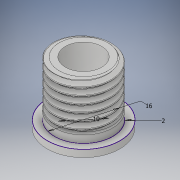
# Autodesk Inventor part: LegScrew
Saved by Autodesk Inventor 2018.2 (Build 222227000, 227)
## iProperties
Created: 2018-03-10
Part Number: LegScrew
Material: Generisch
Document SubType Name: Modeling
Designer: JochenAlt
Density: 1 g/cm^3
Appearance: Vorgabe
Author: JochenAlt
Autodesk Inventor part; units mm, degrees
ref_plane "YZ Plane" through (0, 0, 0) normal (1, 0, 0) x (0, 1, 0)
ref_plane "XZ Plane" through (0, 0, 0) normal (0, 1, 0) x (-1, 0, 0)
ref_plane "XY Plane" through (0, 0, 0) normal (0, 0, 1) x (1, 0, 0)
sketch "Skizze1" plane through (0, 0, 0) normal (0, 0, 1) x (1, 0, 0)
  circle A0 centre (0, 0) radius 5
  circle A1 centre (0, 0) radius 10
  circle A2 centre (0, 0) radius 8
  dimension "d0" = 10
  dimension "d1" = 16
  dimension "d2" = 2
  constraints: 3 centre point, 3 coincident
  measures "d0" diameter of A0
  measures "d1" diameter of A2
  measures "d2" radial gap between concentric circles of A1 A2
extrude "Extrusion1" add sketch "Skizze1" along normal blind 15 contours A2
extrude "Extrusion2" add sketch "Skizze1" against normal blind 2 contours A1 | A2
thread "Gewinde3" size "M16x2" class "6g" standard "ANSI Metric M Profile" length 13
sketch "Skizze9" plane through (0, 0, 15) normal (-1, 0, 0) x (0, 1, 0)
  line L0 (8, 0) -> (8, 13)
  line L1 (8, 13) -> (6.6948, 13)
  line L2 (6.6948, 13) -> (6.6948, 0)
  line L3 (6.6948, 0) -> (8, 0)
  line L4 (0, -2.6) -> (0, 15.6) projected
  constraints: 8 end point
revolve "Umdrehung5" cut sketch "Skizze9" angle 360 about axis through (0, 0, 15) along (0, 0, -1)
sketch "Skizze10" plane through (0, 0, 15) normal (-1, 0, 0) x (0, 1, 0)
  line L0 (8, 0) -> (8, 13)
  line L1 (8, 13) -> (6.6948, 13)
  line L2 (6.6948, 13) -> (6.6948, 0)
  line L3 (6.6948, 0) -> (8, 0)
  line L4 (0, -2.6) -> (0, 15.6) projected
  constraints: 8 end point
revolve "Umdrehung6" add sketch "Skizze10" angle 360 about axis through (0, 0, 15) along (0, 0, -1) separate body
sketch "Skizze8" plane through (0, 0, 15) normal (1, 0, 0) x (0, 0, -1)
  line L0 (-1.1849, -6.8017) -> (-1.0001, -6.8017) construction
  line L1 (0.1847, -7.8934) -> (-0.0001, -8.2136) construction
  line L2 (-2.0001, -8.2136) -> (-2.185, -7.8934) construction
  line L3 (-0.8153, -6.8017) -> (-1.0001, -6.4816) construction
  line L4 (-1.0001, -6.4816) -> (-1.1849, -6.8017) construction
  line L5 (-2.0001, -8.2136) -> (-1.8153, -7.8934) construction
  line L6 (-0.8153, -6.8017) -> (-0.1849, -7.8934)
  line L7 (-2.185, -7.8934) -> (-1.8153, -7.8934) construction
  arc A0 (-2.185, -7.8934) -> (-2.0001, -8.0002) centre (-2.0001, -7.7867) ccw construction
  line L8 (0.1847, -7.8934) -> (-0.1849, -7.8934) construction
  line L9 (-2.0001, -8.2136) -> (-2.0001, -7.8934) construction
  line L10 (-0.0001, -8.2136) -> (-0.0001, -7.8934) construction
  line L11 (-1.0001, -6.4816) -> (-1.0001, -6.695) construction
  line L12 (-2.0001, -8.0002) -> (-0.0001, -8.0002)
  arc A1 (-2.0001, -8.0002) -> (-1.8153, -7.8934) centre (-2.0001, -7.7867) ccw
  line L13 (-0.1849, -7.8934) -> (-0.0001, -8.2136) construction
  line L14 (-1.8153, -7.8934) -> (-1.1849, -6.8017)
  line L15 (-0.0001, -0.0002) -> (-0.0001, 0.0177)
  line L16 (-0.0001, 0.0177) -> (-0.0001, -0.0002)
  line L17 (-0.0001, -0.0002) -> (0.0334, -0.0002)
  arc A2 (-0.1849, -7.8934) -> (-0.0001, -8.0002) centre (-0.0001, -7.7867) ccw
  arc A3 (-0.0001, -8.0002) -> (0.1847, -7.8934) centre (-0.0001, -7.7867) ccw construction
  arc A4 (-1.0001, -6.695) -> (-1.1849, -6.8017) centre (-1.0001, -6.9084) ccw
  arc A5 (-0.8153, -6.8017) -> (-1.0001, -6.695) centre (-1.0001, -6.9084) ccw
  line L18 (-1.0001, -6.695) -> (-1.0001, -6.8017) construction
  line L19 (-1.0001, -6.8017) -> (-0.8153, -6.8017) construction
  dimension "d51" = 60
  dimension "d52" = 0.3202
  dimension "d53" = 0.3202
  dimension "Skizze8_ThreadOffset" = 0
  dimension "Skizze8_MajorRadius" = 8
  dimension "d56" = 2
  dimension "Skizze8_MinorRadius" = 6.6948
  constraints: 40 end point, 12 point on circle, 10 parallel, 8 tangent, 6 centre point, 6 collinear, 2 midpoint, 2 point on line, 1 horizontal, 1 perpendicular, 3 other
  measures "d51" angle of L6 L14
  measures "d52" distance of L3.end L0.end
  measures "d53" distance of L1.end L10.end
  measures "Skizze8_ThreadOffset" distance between parallel lines of L15 L10
  measures "Skizze8_MajorRadius" distance from line of L12 L15.start
  measures "d56" distance from line of L1.end L9
  measures "Skizze8_MinorRadius" distance edge to line of A5 L17
coil "Spirale3" sketch "Skizze8" operation cut axis through (0, 0, 15) along (0, 0, -1) pitch 2.002 turns 8.491508 hand right bodies 2
equation "\"d51\" = d58"
equation "\"d52\" = 0.160083 * Skizze8_Pitch"
equation "\"d53\" = 0.160083 * Skizze8_Pitch"
equation "\"d56\" = Skizze8_Pitch"
equation "\"d16\" = 60deg"
equation "\"Skizze2_Pitch\" = 2.5"
equation "\"d37\" = 60deg"
equation "\"Skizze5_Pitch\" = 3"
equation "\"d58\" = 60deg"
equation "\"Skizze8_Pitch\" = 2"
